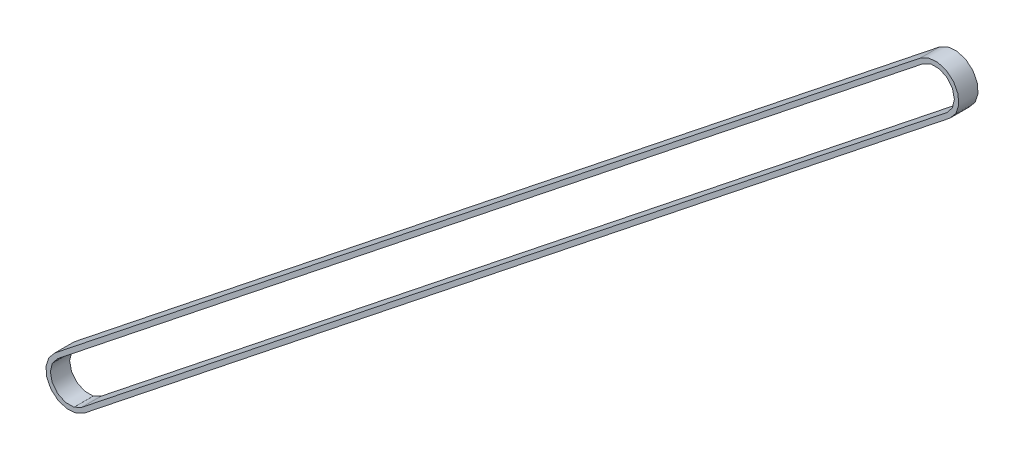
# Autodesk Inventor part: ремень оси x
Saved by Autodesk Inventor 2017 (Build 210142000, 142)
## iProperties
Part Number: ремень оси x
Material: Типовые
Document SubType Name: Modeling
Designer: Max
Mass: 6.13101 g
Surface Area: 108.023 cm^2
Volume: 6.13101 cm^3
Density: 1 g/cm^3
Appearance: Резина — черная — версия 1.1
Author: Max
Autodesk Inventor part; units mm, degrees
ref_plane "YZ Plane" through (0, 0, 0) normal (1, 0, 0) x (0, 1, 0)
ref_plane "XZ Plane" through (0, 0, 0) normal (0, 1, 0) x (-1, 0, 0)
ref_plane "XY Plane" through (0, 0, 0) normal (0, 0, 1) x (1, 0, 0)
sketch "Эскиз1" plane through (0, 0, 0) normal (0, 0, 1) x (1, 0, 0)
  arc A0 (-3.7341, 4.6965) -> (3.7341, -4.6965) centre (0, 0) ccw
  arc A1 (-4.6053, 5.7923) -> (4.6053, -5.7923) centre (0, 0) ccw
  circle A2 centre (269.1802, 214.0185) radius 8.8 construction
  arc A3 (272.9142, 209.3221) -> (265.4461, 218.715) centre (269.1802, 214.0185) ccw
  arc A4 (273.7855, 208.2262) -> (264.5748, 219.8109) centre (269.1802, 214.0185) ccw
  line L0 (264.5748, 219.8109) -> (-4.6053, 5.7923)
  line L1 (-3.7341, 4.6965) -> (265.4461, 218.715)
  line L2 (272.9142, 209.3221) -> (3.7341, -4.6965)
  line L3 (4.6053, -5.7923) -> (273.7855, 208.2262)
  dimension "d0" = 12
  dimension "d1" = 1.4
  dimension "d2" = 12
  dimension "d3" = 1.4
  constraints: 8 end point, 8 point on circle, 5 tangent, 4 centre point, 4 coincident, 3 parallel
  measures "d0" diameter of A0
  measures "d1" radial gap between concentric circles of A1 A0
  measures "d2" diameter of A3
  measures "d3" radial gap between concentric circles of A4 A3
extrude "Выдавливание1" add sketch "Эскиз1" along normal blind 6
